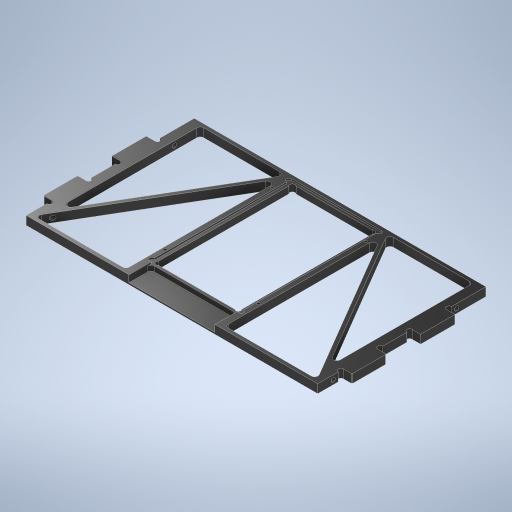
# Autodesk Inventor part: TorsoLowerFrame
Saved by Autodesk Inventor 2024.2 (Build 282272000, 272)
## iProperties
Created: 2024-01-11
Part Number: TorsoLowerFrame
Material: Aluminum 2014-T4
Document SubType Name: Modeling
Designer: Masato Kubotera
Density: 2.8 g/cm^3
Appearance: Glossy - Black
Vendor: meviy
Mass: 47.2837 g
Surface Area: 169.328 cm^2
Volume: 16.887 cm^3
Author: Masato Kubotera
Autodesk Inventor part; units mm, degrees
ref_plane "YZ Plane" through (0, 0, 0) normal (1, 0, 0) x (0, 1, 0)
ref_plane "XZ Plane" through (0, 0, 0) normal (0, 1, 0) x (-1, 0, 0)
ref_plane "XY Plane" through (0, 0, 0) normal (0, 0, 1) x (1, 0, 0)
sketch "Sketch1" plane through (0, 0, 0) normal (0, 0, 1) x (1, 0, 0)
  line L0 (-53, -85) -> (45, -85)
  line L1 (45, 85) -> (-53, 85) construction
  line L2 (0, -85) -> (0, 85) construction
  line L3 (-53, 0) -> (45, 0)
  line L4 (10, 90) -> (30, 90)
  line L5 (10, 90) -> (10, 85)
  arc A0 (7, 85) -> (10, 85) centre (8.5, 85) ccw
  line L6 (45, 85) -> (45, -85)
  line L7 (-53, -85) -> (-53, 85)
  line L8 (31.85, -25.8) -> (-50.75, -25.8) construction
  line L9 (-50.75, -25.8) -> (-50.75, 25.8) construction
  line L10 (-50.75, 25.8) -> (31.85, 25.8) construction
  line L11 (31.85, 25.8) -> (31.85, -25.8) construction
  line L12 (31.85, -25.8) -> (-50.75, 25.8) construction
  line L13 (-50.75, -25.8) -> (31.85, 25.8) construction
  line L14 (32.1, -26.05) -> (-51, -26.05)
  line L15 (-51, -26.05) -> (-51, 26.05)
  line L16 (-51, 26.05) -> (32.1, 26.05)
  line L17 (32.1, 26.05) -> (32.1, -26.05)
  line L18 (32.1, -26.05) -> (-51, 26.05) construction
  line L19 (-51, -26.05) -> (32.1, 26.05) construction
  line L20 (-49.5, 24.3) -> (30.6, 24.3)
  line L21 (30.6, 24.3) -> (30.6, -24.3)
  line L22 (30.6, -24.3) -> (-49.5, -24.3)
  line L23 (-49.5, -24.3) -> (-49.5, 24.3)
  line L24 (-49.5, 24.3) -> (30.6, -24.3) construction
  line L25 (30.6, 24.3) -> (-49.5, -24.3) construction
  line L26 (43, 30.8) -> (43, 79.1635)
  line L27 (39.9853, 80.887) -> (-42.1573, 32.5235)
  line L28 (-41.1426, 28.8) -> (41, 28.8)
  line L29 (-47.9853, 31.413) -> (27.3635, 75.7765)
  line L30 (26.3488, 79.5) -> (-49, 79.5)
  line L31 (-51, 77.5) -> (-51, 33.1365)
  line L32 (45, 27.3) -> (-53, 27.3) construction
  line L33 (-53, 27.3) -> (45, 85) construction
  arc A1 (41, 28.8) -> (43, 30.8) centre (41, 30.8) ccw
  arc A2 (43, 79.1635) -> (39.9853, 80.887) centre (41, 79.1635) ccw
  arc A3 (-42.1573, 32.5235) -> (-41.1426, 28.8) centre (-41.1426, 30.8) ccw
  arc A4 (-51, 33.1365) -> (-47.9853, 31.413) centre (-49, 33.1365) ccw
  arc A5 (27.3635, 75.7765) -> (26.3488, 79.5) centre (26.3488, 77.5) ccw
  arc A6 (-49, 79.5) -> (-51, 77.5) centre (-49, 77.5) ccw
  arc A7 (32.1, 26.05) -> (29.1, 26.05) centre (30.6, 26.05) ccw
  line L34 (32.1, 25.05) -> (45, 25.05)
  arc A8 (30.6, 22.1787) -> (28.4787, 24.3) centre (29.5393, 23.2393) ccw
  arc A9 (-47.3787, 24.3) -> (-49.5, 22.1787) centre (-48.4393, 23.2393) ccw
  arc A10 (-48, 26.05) -> (-51, 26.05) centre (-49.5, 26.05) ccw
  circle A11 centre (21.85, 27.3) radius 1.5 construction
  circle A12 centre (21.85, 27.3) radius 1 construction
  line L35 (-9.45, -25.8) -> (-9.45, 25.7819) construction
  circle A13 centre (-40.75, 27.3) radius 1.5 construction
  circle A14 centre (-40.75, 27.3) radius 1 construction
  circle A15 centre (21.85, 27.3) radius 2.5 construction
  circle A16 centre (-40.75, 27.3) radius 2.5 construction
  line L36 (20, 90) -> (20, 85) construction
  line L37 (30, 90) -> (30, 85)
  arc A17 (30, 85) -> (33, 85) centre (31.5, 85) ccw
  line L38 (45, 85) -> (33, 85)
  line L39 (-10, 90) -> (-30, 90)
  line L40 (-10, 90) -> (-10, 85)
  arc A18 (-10, 85) -> (-7, 85) centre (-8.5, 85) ccw
  line L41 (-20, 90) -> (-20, 85) construction
  line L42 (-30, 90) -> (-30, 85)
  arc A19 (-33, 85) -> (-30, 85) centre (-31.5, 85) ccw
  line L43 (7, 85) -> (-7, 85)
  line L44 (-33, 85) -> (-53, 85)
  line L45 (36, 85) -> (36, 79) construction
  line L46 (-36, 85) -> (-36, 79) construction
  point P0 (0, 0)
  point P1 (50, -85)
  point P2 (-47, 0)
  point P3 (-9.45, 0)
  point P4 (-51, 0)
  point P5 (32.1, 0)
  point P6 (-24.777, 28.8)
  point P7 (-49.5, 0)
  point P8 (30.6, 0)
  dimension "d1" = 170
  dimension "d2" = 1.5
  dimension "d3" = 5
  dimension "d55" = 82.6
  dimension "d56" = 51.6
  dimension "d57" = 0.25
  dimension "d58" = 0.25
  dimension "d62" = 2
  dimension "d63" = 2
  dimension "d66" = 2
  dimension "d71" = 1
  dimension "d81" = 3
  dimension "d82" = 2
  dimension "d85" = 1.5
  dimension "d86" = 1.5
  dimension "d94" = 10
  dimension "d95" = 5
  dimension "d97" = 2
  dimension "d99" = 6
  dimension "d100" = 6
  dimension "d101" = 98
  dimension "d102" = 20
  dimension "d103" = 20
  dimension "d104" = 45
  dimension "d105" = 5.5
  constraints: 96 end point, 30 point on circle, 25 point on line, 20 centre point, 19 symmetric about line, 16 tangent, 11 midpoint, 9 equal radius, 9 horizontal, 8 parallel, 7 vertical, 5 coincident, 3 collinear, 3 perpendicular, 8 other
  measures "d1" distance of L1.start L0.end
  measures "d2" radius of A0
  measures "d3" distance of L4.start L5.end
  measures "d55" distance of L9.end L10.end
  measures "d56" distance of L8.end L9.end
  measures "d57" distance between parallel lines of L16 L10
  measures "d58" distance between parallel lines of L15 L9
  measures "d62" radius of A1
  measures "d63" distance between parallel lines of L27 L29
  measures "d66" distance between parallel lines of L6 L26
  measures "d71" distance of A7.start L34.start
  measures "d81" diameter of A11
  measures "d82" diameter of A12
  measures "d85" distance between parallel lines of L10 L20
  measures "d86" distance between parallel lines of L21 L17
  measures "d94" horizontal distance of L10.end A11.centre
  measures "d95" diameter of A15
  measures "d97" distance between parallel lines of L7 L31
  measures "d99" distance of L45.start L45.end
  measures "d100" distance between parallel lines of L37 L45
  measures "d101" distance between parallel lines of L7 L6
  measures "d102" distance of L4.start L4.end
  measures "d103" distance between parallel lines of L40 L5
  measures "d104" distance between parallel lines of L6 L2
  measures "d105" distance between parallel lines of L44 L30
extrude "Extrusion1" add sketch "Sketch1" against normal blind 5 contours L7 L44 A19 L42 L39 L40 A18 L43 A0 L5 L4 L37 A17 L38 L6 L34 L17 A7 L16 A10 L15 L3 | L3 L17 L34 L6 | L15 L16 L17 L3 L21 A8 L20 A9 L23 | A10 L16 | L16 A7
extrude "Extrusion2" cut sketch "Sketch1" against normal blind 1 contours L15 L16 L17 L3 L21 A8 L20 A9 L23 | A10 L16 | L16 A7
extrude "Extrusion3" cut sketch "Sketch1" against normal blind 4 contours L3 L17 L34 L6
hole "Hole5" at (21.85, 27.3, 0) at (-40.75, 27.3, 0) direction (0, 0, -1) diameter 1.567 end through all thread size "M2x0.4" class "6H" standard "ANSI Metric M Profile"
sketch "Sketch6" plane through (33, 85, 0) normal (0, 1, 0) x (1, 0, 0)
  line L0 (0, 5) -> (12, 5) projected
  line L1 (3, 5) -> (3, 0)
  line L2 (12, 0) -> (0, 0) projected
  line L3 (-86, 5) -> (-66, 5) projected
  line L4 (-69, 5) -> (-69, 0)
  line L5 (-66, 0) -> (-86, 0) projected
  point P0 (-33, 0)
  point P1 (3, 0)
  point P2 (-69, 0)
  point P3 (3, 2.5)
  point P4 (-69, 2.5)
  constraints: 4 end point, 2 midpoint, 2 point on line, 2 vertical
hole "Hole6" at (36, 85, -2.5) at (-36, 85, -2.5) direction (0, -1, 0) diameter 2.459 depth 10 thread size "M3x0.5" class "6H" standard "ANSI Metric M Profile"
ref_plane "Work Plane1" through (-9.45, 0, -5) normal (1, 0, 0) x (0, 0, -1)
chamfer "Chamfer1" distance 0.5 angle 45 2 edges at (30, 90, -2.5) (10, 90, -2.5)
fillet "Fillet1" radius 2 1 edges at (32.1, 25.05, -2.5)
mirror "Mirror5" about plane through (0, 0, 0) normal (0, 1, 0)
body "Solid1"
